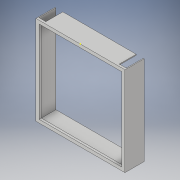
# Autodesk Inventor part: tec_holder
Saved by Autodesk Inventor 2018 (Build 220112000, 112)
## iProperties
Created: 2018-02-10
Part Number: tec_holder
Material: Generic
Document SubType Name: Modeling
Designer: Benedikt
Density: 1 g/cm^3
Appearance: Default
Author: Benedikt
Autodesk Inventor part; units mm, degrees
ref_plane "YZ Plane" through (0, 0, 0) normal (1, 0, 0) x (0, 1, 0)
ref_plane "XZ Plane" through (0, 0, 0) normal (0, 1, 0) x (-1, 0, 0)
ref_plane "XY Plane" through (0, 0, 0) normal (0, 0, 1) x (1, 0, 0)
sketch "Sketch1" plane through (0, 0, 0) normal (0, 1, 0) x (-1, 0, 0)
  line L0 (-19, 19) -> (19, 19)
  line L1 (19, 19) -> (19, -19)
  line L2 (19, -19) -> (-19, -19)
  line L3 (-19, -19) -> (-19, 19)
  line L4 (-19, 19) -> (19, -19) construction
  line L5 (19, 19) -> (-19, -19) construction
  line L6 (-20.5, 20.5) -> (20.5, 20.5)
  line L7 (20.5, 20.5) -> (20.5, -20.5)
  line L8 (20.5, -20.5) -> (-20.5, -20.5)
  line L9 (-20.5, -20.5) -> (-20.5, 20.5)
  line L10 (-20.5, 20.5) -> (20.5, -20.5) construction
  line L11 (20.5, 20.5) -> (-20.5, -20.5) construction
  point P0 (0, 0)
  dimension "d0" = 38
  dimension "d1" = 38
  dimension "d2" = 41
  dimension "d3" = 41
  constraints: 24 end point, 4 midpoint, 4 parallel, 2 horizontal, 2 perpendicular
  measures "d0" distance of L1.end L2.end
  measures "d1" distance of L0.end L1.end
  measures "d2" distance of L7.end L8.end
  measures "d3" distance of L6.end L7.end
extrude "Extrusion1" add sketch "Sketch1" along normal blind 1
sketch "Sketch2" plane through (0, 1, 0) normal (0, 1, 0) x (1, 0, 0)
  line L0 (-20.5, -20.5) -> (20.5, -20.5) projected
  line L1 (-20.5, 20.5) -> (20.5, 20.5)
  line L2 (20.5, 20.5) -> (20.5, -20.5)
  line L3 (20.5, -20.5) -> (-20.5, -20.5)
  line L4 (-20.5, -20.5) -> (-20.5, 20.5)
  line L5 (-20.5, 20.5) -> (20.5, -20.5) construction
  line L6 (20.5, 20.5) -> (-20.5, -20.5) construction
  line L7 (-20.1, 20.1) -> (20.1, 20.1)
  line L8 (20.1, 20.1) -> (20.1, -20.1)
  line L9 (20.1, -20.1) -> (-20.1, -20.1)
  line L10 (-20.1, -20.1) -> (-20.1, 20.1)
  line L11 (-20.1, 20.1) -> (20.1, -20.1) construction
  line L12 (20.1, 20.1) -> (-20.1, -20.1) construction
  point P0 (0, 0)
  dimension "d6" = 40.2
  constraints: 24 end point, 4 midpoint, 4 parallel, 2 horizontal, 2 perpendicular, 1 point on line
  measures "d6" distance of L8.end L9.end
extrude "Extrusion2" add sketch "Sketch2" along normal blind 7.8
sketch "Sketch3" plane through (-20.5, 0, 20.5) normal (0, 0, 1) x (1, 0, 0)
  point P0 (20.5, 0)
sketch "Sketch4" plane through (20.1, 1, 20.1) normal (0, 0, -1) x (-1, 0, 0)
  line L0 (0, 0) -> (40.2, 0) projected
  line L1 (40.2, 0) -> (0, 0) projected
  line L2 (39.1, 0) -> (1.1, 0) projected
  line L3 (1.1, 0) -> (39.1, 0) projected
  line L4 (40.2, 0) -> (0, 0) projected
  line L5 (0, 7.8) -> (40.2, 7.8) projected
  line L6 (0, 0) -> (3.2, 0)
  line L7 (3.2, 0) -> (3.2, 7.8)
  line L8 (3.2, 7.8) -> (0, 7.8)
  line L9 (0, 7.8) -> (0, 0)
  line L10 (40.2, 0) -> (37, 0)
  line L11 (37, 0) -> (37, 7.8)
  line L12 (37, 7.8) -> (40.2, 7.8)
  line L13 (40.2, 7.8) -> (40.2, 0)
  point P0 (20.1, -1)
  dimension "d9" = 3.2
  dimension "d10" = 3.2
  constraints: 16 end point, 4 parallel, 2 horizontal, 2 perpendicular, 2 point on line
  measures "d9" distance of L8.end L7.end
  measures "d10" distance of L11.end L12.end
extrude "Extrusion3" cut sketch "Sketch4" against normal blind 7.8 contours L9 L5 L7 L0 | L11 L5 L13 L0
body "Solid1"
